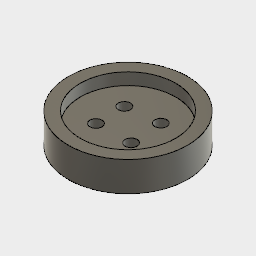
FPROJ_6_Czw (Autodesk Fusion 360 design; units mm, degrees)
Autodesk Fusion 360 part; units mm, degrees
sketch "草图1" plane through (0, 0, 0) normal (0, 1, 0) x (1, 0, 0)
  circle A0 centre (0, 0) radius 10
  circle A1 centre (0, 0) radius 8
  dimension "d1" = 2
extrude "拉伸1" add sketch "草图1" along normal blind 3 contours A1 makes body 1
extrude "拉伸2" add sketch "草图1" along normal blind 5 separate body makes body 2
cylinder "圆柱体基本要素1" add diameter 2 height 20 placed x (1, 0, 0) y (0, 0, -1) z (0, 1, 0) at (11, 0, -24) separate body makes body 3
move_body "移动1" bodies 3 to x (1, 0, 0) y (0, 1, 0) z (0, 0, 1) at (-11.0071, 0, 23.9842)
pattern_linear "R-阵列1" count 2 spacing 6 along (1, 0, 0) count 2 spacing 4 along (0, 0, 1) of bodies 3 makes body 4 at (6.9879, 13.3333, 0.0837) makes body 5 at (0.9917, 6.6667, 4.034) makes body 6 at (6.9879, 13.3333, 4.0837)
move_body "移动2" bodies 3 to x (1, 0, 0) y (0, 1, 0) z (0, 0, 1) at (-2.932, 0.1861, -2.3224)
move_body "移动3" bodies 4 to x (1, 0, 0) y (0, 1, 0) z (0, 0, 1) at (-3.4385, 0.2252, -2.9374)
move_body "移动4" bodies 5 to x (1, 0, 0) y (0, 1, 0) z (0, 0, 1) at (-3.0212, 0.1585, -1.3655)
move_body "移动5" bodies 6 to x (1, 0, 0) y (0, 1, 0) z (0, 0, 1) at (-3.0832, 0.2183, -1.5885)
move_body "移动6" bodies 5 to x (1, 0, 0) y (0, 1, 0) z (0, 0, 1) at (0.1848, 0, -0.0924)
move_body "移动7" bodies 3 to x (1, 0, 0) y (0, 1, 0) z (0, 0, 1) at (0, -10, 0)
move_body "移动8" bodies 4 to x (1, 0, 0) y (0, 1, 0) z (0, 0, 1) at (0, -11, 0)
move_body "移动9" bodies 6 to x (1, 0, 0) y (0, 1, 0) z (0, 0, 1) at (0, -6, 0)
move_body "移动10" bodies 5 to x (1, 0, 0) y (0, 1, 0) z (0, 0, 1) at (0, -7, 0)
combine "合并1" operation cut target body 1 tool bodies 5 3 6 4
combine "合并2" operation add target body 1 tool bodies 2
